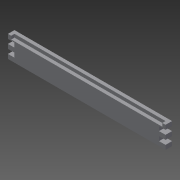
# Autodesk Inventor part: top_cover_side
Saved by Autodesk Inventor 2014 SP1 (Build 180222100, 222)
## iProperties
Created: 2014-02-23
Part Number: top_cover_side
Material: Wood (Birch)
Document SubType Name: Modeling
Designer: Chris
Density: 0.55 g/cm^3
Appearance: Birch - Natural Polished
Mass: 274.136 g
Surface Area: 795.765 cm^2
Volume: 498.429 cm^3
Author: Chris
Autodesk Inventor part; units mm, degrees
ref_plane "YZ Plane" through (0, 0, 0) normal (1, 0, 0) x (0, 1, 0)
ref_plane "XZ Plane" through (0, 0, 0) normal (0, 1, 0) x (-1, 0, 0)
ref_plane "XY Plane" through (0, 0, 0) normal (0, 0, 1) x (1, 0, 0)
sketch "Sketch1" plane through (0, 0, 0) normal (0, 0, 1) x (1, 0, 0)
  line L0 (293.6875, 89.6306) -> (523.875, 89.6306)
  line L1 (523.875, 89.6306) -> (523.875, 26.1306)
  line L2 (523.875, 26.1306) -> (293.6875, 26.1306)
  line L3 (293.6875, 89.6306) -> (293.6875, 76.9306)
  line L4 (293.6875, 76.9306) -> (274.6375, 76.9306)
  line L5 (274.6375, 76.9306) -> (274.6375, 64.2306)
  line L6 (274.6375, 64.2306) -> (293.6875, 64.2306)
  line L7 (293.6875, 64.2306) -> (293.6875, 51.5306)
  line L8 (293.6875, 51.5306) -> (274.6375, 51.5306)
  line L9 (274.6375, 51.5306) -> (274.6375, 38.8306)
  line L10 (274.6375, 38.8306) -> (293.6875, 38.8306)
  line L11 (293.6875, 38.8306) -> (293.6875, 26.1306)
  line L12 (293.6875, 76.9306) -> (312.7375, 76.9306)
  line L13 (312.7375, 76.9306) -> (312.7375, 64.2306)
  line L14 (312.7375, 64.2306) -> (293.6875, 64.2306)
  line L15 (293.6875, 51.5306) -> (312.7375, 51.5306)
  line L16 (312.7375, 51.5306) -> (312.7375, 38.8306)
  line L17 (312.7375, 38.8306) -> (293.6875, 38.8306)
  point P0 (0, 0)
  dimension "d4" = 63.5
  dimension "d17" = 230.1875
  dimension "d18" = 19.05
  dimension "d19" = 12.7
  dimension "d20" = 12.7
  dimension "d21" = 12.7
  dimension "d22" = 12.7
  dimension "d23" = 12.7
  dimension "d24" = 0
  dimension "d28" = 0
  constraints: 36 end point, 7 perpendicular, 4 parallel, 4 symmetric about line, 1 horizontal
  measures "d4" distance of L0.end L1.end
  measures "d17" distance of L0.start L0.end
  measures "d18" distance of L3.end L4.end
  measures "d19" distance of L0.start L3.end
  measures "d20" distance of L4.end L5.end
  measures "d21" distance of L6.end L7.end
  measures "d22" distance of L8.end L9.end
  measures "d23" distance of L10.end L2.end
  measures "d24" distance between parallel lines of L11 L7
  measures "d28" distance between parallel lines of L7 L3
extrude "Extrusion4" add sketch "Sketch1" along normal blind 19.05 contours L0 L1 L2 L11 L17 L16 L15 L7 L14 L13 L12 L3
mirror "Mirror2" about plane through (523.875, 26.1306, 0) normal (1, 0, 0) of "Extrusion4"
sketch "Sketch4" plane through (293.6875, 89.6306, 19.05) normal (0, 1, 0) x (1, 0, 0)
  line L0 (0, 19.05) -> (0, 0) projected
  line L1 (0, 0) -> (460.375, 0) projected
  line L2 (460.375, 19.05) -> (460.375, 0) projected
  line L3 (9.525, 0) -> (450.85, 0)
  line L4 (450.85, 0) -> (450.85, 9.525)
  line L5 (450.85, 9.525) -> (9.525, 9.525)
  line L6 (9.525, 9.525) -> (9.525, 0)
  point P0 (-293.6875, 19.05)
  dimension "d32" = 9.525
  dimension "d34" = 9.525
  constraints: 8 end point, 2 parallel, 1 horizontal, 1 perpendicular, 1 point on line
  measures "d32" distance between parallel lines of L0 L6
  measures "d34" distance between parallel lines of L2 L4
extrude "Extrusion5" cut sketch "Sketch4" against normal blind 9.525
body "Solid2"
